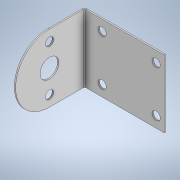
# Autodesk Inventor part: wheel_base
Saved by Autodesk Inventor 2022 (Build 260153000, 153)
## iProperties
Created: 2023-03-16
Part Number: wheel_base
Material: 一般
Document SubType Name: Sheet Metal
Designer: JOU
Density: 1 g/cm^3
Sheet Metal Rule: 預設 mm (_M)
Appearance: 預設
Author: JOU
Autodesk Inventor part; units mm, degrees
ref_plane "YZ Plane" through (0, 0, 0) normal (1, 0, 0) x (0, 1, 0)
ref_plane "XZ Plane" through (0, 0, 0) normal (0, 1, 0) x (-1, 0, 0)
ref_plane "XY Plane" through (0, 0, 0) normal (0, 0, 1) x (1, 0, 0)
sketch "草圖1" plane through (0, 0, 0) normal (0, 1, 0) x (-1, 0, 0)
  line L0 (29.5719, -39.0966) -> (29.5719, -13.0966)
  line L1 (29.5719, -39.0966) -> (-0.4281, -39.0966)
  point P0 (0, 0)
  dimension "d0" = 26
  dimension "d2" = 90
  dimension "d3" = 30
  measures "d0" distance of L0.start L0.end
  measures "d2" angle of L1 L0
  measures "d3" distance of L0.start L1.end
contour flange "輪廓線凸緣1" sketch "草圖1" thickness 0.5 bend radius 0.5 width 25 along (0, 1, 0) mid plane no both sides no wall seen from (-29.5719, 0, -26.0966) lies toward (1, 0, 0) curves L0 L1
bend "折彎1"
corner "轉角1"
sketch "草圖2" plane through (-29.0719, 0, -13.0966) normal (1, 0, 0) x (0, 0, -1)
  circle A0 centre (12.5, 12.5) radius 12.5
  line L0 (0, 25) -> (25, 25) projected
  line L1 (0, 0) -> (0, 25) projected
  line L2 (0, 0) -> (25, 0) projected
  point P0 (-13.0966, 0)
  point P1 (0, 12.5)
  point P2 (12.5, 25)
  point P3 (12.5, 0)
  dimension "d15" = 25
  constraints: 2 tangent, 1 centre point
  measures "d15" diameter of A0
extrude "擠出1" cut sketch "草圖2" against normal up to surface (0.5 mm away) contours A0 L1 L0 | L2 L1 A0
sketch "草圖3" plane through (-29.0719, 0, -38.0966) normal (1, 0, 0) x (0, 0, -1)
  arc A0 (-12.5, 25) -> (-12.5, 0) centre (-12.5, 12.5) ccw projected
  circle A1 centre (-12.5, 21) radius 1.5
  circle A2 centre (-12.5, 4) radius 1.5
  point P0 (-38.0966, 0)
  dimension "d18" = 3
  dimension "d19" = 17
  dimension "d20" = 8.5
  dimension "d21" = 3
  constraints: 2 centre point, 2 vertical alignment
  measures "d18" diameter of A1
  measures "d19" distance of A2.centre A1.centre
  measures "d20" distance of A0.centre A1.centre
  measures "d21" diameter of A2
extrude "擠出2" cut sketch "草圖3" against normal up to surface (0.5 mm away)
sketch "草圖4" plane through (0.4281, 0, -38.5966) normal (0, 0, 1) x (1, 0, 0)
  circle A0 centre (-23, 21) radius 1.5
  circle A1 centre (-3, 21) radius 1.5
  circle A2 centre (-23, 4) radius 1.5
  circle A3 centre (-3, 4) radius 1.5
  line L0 (0, 0) -> (0, 25) projected
  line L1 (-3, 21) -> (-3, 4)
  line L2 (-3, 12.5) -> (-13.1347, 12.5)
  line L3 (-29, 25) -> (0, 25) projected
  point P0 (-0.4281, 0)
  dimension "d24" = 20
  dimension "d25" = 3
  dimension "d26" = 3
  dimension "d27" = 3
  dimension "d28" = 3
  dimension "d29" = 17
  dimension "d30" = 3
  dimension "d31" = 12.5
  constraints: 4 centre point, 4 end point, 2 horizontal alignment, 2 vertical alignment, 1 horizontal, 1 midpoint, 1 vertical
  measures "d24" distance of L1.start A0.centre
  measures "d25" diameter of A1
  measures "d26" diameter of A0
  measures "d27" diameter of A2
  measures "d28" diameter of A3
  measures "d29" distance of A2.centre A0.centre
  measures "d30" distance from line of L0 L1.start
  measures "d31" distance between parallel lines of L3 L2
extrude "擠出3" cut sketch "草圖4" against normal up to surface (0.5 mm away)
sketch "草圖5" plane through (-29.0719, 0, -38.0966) normal (1, 0, 0) x (0, 0, -1)
  arc A0 (-12.5, 25) -> (-12.5, 0) centre (-12.5, 12.5) ccw projected
  circle A1 centre (-12.5, 12.5) radius 3.5
  point P0 (-38.0966, 0)
  dimension "d34" = 7
  constraints: 1 centre point, 1 coincident
  measures "d34" diameter of A1
extrude "擠出4" cut sketch "草圖5" against normal up to surface (0.5 mm away)
equation "\"d4\" = 厚度"
equation "\"d5\" = 折彎離隙寬度"
equation "\"d6\" = 折彎離隙深度"
equation "\"d7\" = 最小剩餘"
equation "\"d8\" = 轉移半徑"
equation "\"d10\" = 折彎半徑"
equation "\"d12\" = 轉角離隙大小"
equation "\"d13\" = 間隙大小"
equation "\"d14\" = Jacobi半徑大小"
equation "\"折彎半徑\" = 厚度"
equation "\"折彎離隙寬度\" = 厚度"
equation "\"折彎離隙深度\" = 0.5 * 厚度"
equation "\"轉角離隙大小\" = 4 * 厚度"
equation "\"最小剩餘\" = 2 * 厚度"
equation "\"轉移半徑\" = 折彎半徑"
equation "\"Jacobi半徑大小\" = 折彎半徑"
equation "\"間隙大小\" = 厚度"
equation "\"厚度\" = 0.5"
